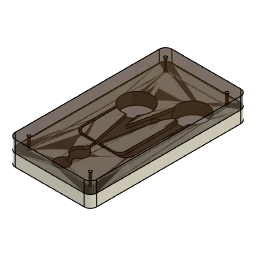
Exhaust_PEEP v7 (Autodesk Fusion 360 design; units mm, degrees)
Autodesk Fusion 360 part; units mm, degrees
sketch "Channels" plane through (0, 0, 0) normal (0, 0, 1) x (1, 0, 0)
  line L0 (0, 0) -> (46.5, 0)
  line L1 (46.5, 0) -> (46.5, 83)
  line L2 (46.5, 83) -> (0, 83)
  line L3 (0, 83) -> (0, 0)
  line L4 (27.5, -7) -> (27.5, 90) construction
  line L5 (10.6, 83) -> (10.6, 31.27) construction
  line L6 (46.5, 25.27) -> (16.6, 25.27) construction
  arc A0 (10.6, 31.27) -> (16.6, 25.27) centre (16.6, 31.27) ccw construction
  arc A1 (9.83, 31.27) -> (16.6, 24.5) centre (16.6, 31.27) ccw
  arc A2 (11.37, 31.27) -> (16.6, 26.04) centre (16.6, 31.27) ccw
  line L7 (27.5, 48.6) -> (34.1243, 80.3757)
  line L8 (27.5, 48.6) -> (46.5, 48.6) construction
  line L9 (27.5, 48.6) -> (25.0136, 60.5271)
  line L10 (25.8031, 26.04) -> (19.3855, 56.8243)
  line L11 (27.5, 17.9) -> (28.8759, 24.5) construction
  line L12 (29.1969, 26.04) -> (33.9, 48.6) construction
  line L13 (28.35, 24.5) -> (28.35, 21)
  line L14 (26.65, 24.5) -> (26.65, 21)
  arc A3 (28.35, 21) -> (30.6235, 17.0635) centre (32.8947, 21) ccw
  arc A4 (24.3765, 17.0635) -> (26.65, 21) centre (22.1053, 21) ccw
  line L15 (39.7, 26.04) -> (29.1969, 26.04)
  line L16 (25.8031, 26.04) -> (16.6, 26.04)
  line L17 (39.7, 24.5) -> (28.35, 24.5)
  line L18 (26.65, 24.5) -> (16.6, 24.5)
  line L19 (11.37, 57.9106) -> (11.37, 31.27)
  line L20 (9.83, 59.002) -> (9.83, 31.27)
  arc A5 (25.0136, 60.5271) -> (9.83, 59.002) centre (16.69, 67.05) ccw
  arc A6 (11.37, 57.9106) -> (19.3855, 56.8243) centre (16.69, 67.05) ccw
  circle A7 centre (16.69, 67.05) radius 7.5 construction
  line L21 (32.5, 0) -> (32.5, 7.9)
  line L22 (22.5, 0) -> (22.5, 7.9)
  arc A8 (24.3765, 17.0635) -> (22.5, 7.9) centre (27.5, 11.65) ccw
  arc A9 (22.5, 7.9) -> (27.5, 5.4) centre (27.5, 11.65) ccw construction
  arc A10 (27.5, 5.4) -> (32.5, 7.9) centre (27.5, 11.65) ccw construction
  arc A11 (32.5, 7.9) -> (30.6235, 17.0635) centre (27.5, 11.65) ccw
  line L23 (46.5, 29.62) -> (39.7, 29.62)
  line L24 (39.7, 20.92) -> (46.5, 20.92)
  line L25 (46.5, 20.92) -> (46.5, 29.62)
  line L26 (39.7, 29.62) -> (39.7, 26.04)
  line L27 (39.7, 24.5) -> (39.7, 20.92)
  line L28 (39.7, 25.27) -> (39.7, 24.5)
  line L29 (39.7, 26.04) -> (39.7, 25.27)
  arc A12 (41.7025, 72.7975) -> (36.748, 62.2613) centre (61.3232, 57.1381) ccw
  line L30 (29.1969, 26.04) -> (36.748, 62.2613)
  line L31 (39.4202, 75.0798) -> (41.0713, 83) construction
  line L32 (36.748, 62.2613) -> (39.4202, 75.0798) construction
  line L33 (46.5, 68) -> (41.7025, 72.7975)
  line L34 (34.1243, 80.3757) -> (31.5, 83)
  line L35 (39.4202, 75.0798) -> (34.1243, 80.3757)
  line L36 (41.7025, 72.7975) -> (39.4202, 75.0798)
  line L37 (34.1243, 80.3757) -> (34.6713, 83) construction
  line L38 (42.75, 29.62) -> (42.75, 71.75) construction
  arc A13 (30.6235, 17.0635) -> (27.5, 17.9) centre (27.5, 11.65) ccw construction
  arc A14 (24.3765, 17.0635) -> (30.6235, 17.0635) centre (27.5, 11.65) ccw
  arc A15 (27.5, 17.9) -> (24.3765, 17.0635) centre (27.5, 11.65) ccw construction
  circle A16 centre (16.69, 67.05) radius 11.125 construction
  dimension "d1" = 83
  dimension "d2" = 46.5
  dimension "d3" = 19
  dimension "d6" = 6
  dimension "d7" = 10.6
  dimension "d8" = 25.27
  dimension "d11" = 12.5
  dimension "d12" = 12.85
  dimension "d13" = 34.4
  dimension "d14" = 12.6
  dimension "d16" = 3.3939
  dimension "d17" = 0.85
  dimension "d20" = 21.15
  dimension "d21" = 16.69
  dimension "d22" = 15.95
  dimension "d23" = 0.77
  dimension "d24" = 0.77
  dimension "d25" = 11.776
  dimension "d26" = 15
  dimension "d27" = 5
  dimension "d28" = 8.7
  dimension "d29" = 6.8
  dimension "d30" = 15
  dimension "d31" = 15
  dimension "d32" = 37
  dimension "d33" = 2.7
  dimension "d34" = 1.54
  dimension "d35" = 1.7
  dimension "d36" = 6.2653
  dimension "d37" = 3.75
  dimension "d38" = 3.5
  dimension "d65" = 22.25
  constraint horizontal L0
  constraint vertical L1
  constraint horizontal L2
  constraint vertical L3
  constraint coincident L0.start L3.end
  constraint perpendicular L2 L4
  constraint perpendicular L2 L5
  constraint coincident L1 L6.start
  constraint coincident L5 L5.start
  constraint coincident L2 L5.start
  constraint tangent L6 A0
  constraint tangent L5 A0
  constraint coincident L4 A8.centre
  constraint coincident L4 L7.start
  constraint coincident L2 L37.end
  constraint coincident L4 L11.start
  constraint perpendicular L4 L8
  constraint coincident L12.end L8
  constraint coincident L2 L31.end
  constraint parallel L11 L30
  constraint parallel L7 L30
  constraint symmetric L4 L7.start L8.start
  constraint coincident L11.end L17
  constraint collinear L11 L12
  constraint coincident L10.start L15
  constraint perpendicular L13 L17
  constraint symmetric L4 L13.start L14.start
  constraint tangent L13 A3
  constraint coincident A3.end A8
  constraint symmetric L4 A3.end A4.start
  constraint symmetric L4 L13.end L14.end
  constraint symmetric L4 A3 A4
  constraint parallel L6 L15
  constraint concentric A0 A2
  constraint tangent A2 L15
  constraint collinear L15 L16
  constraint parallel L6 L17
  constraint concentric A0 A1
  constraint tangent A1 L17
  constraint collinear L17 L18
  constraint coincident A3 A11.end
  constraint coincident A4 A8.start
  constraint coincident L19.start A5
  constraint tangent A1 L20
  constraint concentric A5 A6
  constraint concentric A6 A7
  constraint coincident L1 L8.end
  constraint coincident L0 L21.start
  constraint coincident L21.end A8
  constraint perpendicular L0 L21
  constraint symmetric L4 L21.start L22.start
  constraint symmetric L4 L21.end L22.end
  constraint coincident L4 A9.end
  constraint concentric A8 A10
  constraint concentric A8 A9
  constraint concentric A10 A13
  constraint concentric A10 A11
  constraint horizontal L23
  constraint vertical L26
  constraint horizontal L24
  constraint vertical L25
  constraint coincident L1 L23.start
  constraint symmetric L6 L23 L24
  constraint coincident L17.start L26
  constraint coincident L6 L28.start
  constraint vertical L29
  constraint parallel L9 L10
  constraint coincident L1 L33.start
  constraint coincident L2 L34.end
  constraint tangent A12 L30
  constraint parallel L30 L37
  constraint collinear L33 L36
  constraint collinear L33 L34
  constraint coincident L33 L38.end
  constraint perpendicular L6 L38
  constraint coincident L23 L38.start
  constraint tangent A3 A11
  constraint concentric A13 A14
  constraint concentric A13 A15
  constraint concentric A5 A16
  measures "d1" distance of L0.start L2.end
  measures "d2" distance of L0.start L0.end
  measures "d3" horizontal distance of L0.end L4.start
  measures "d6" radius of A0
  measures "d7" distance of L3 L5
  measures "d8" distance of L0 L6
  measures "d11" diameter of A8
  measures "d12" distance of A8.centre L17
  measures "d13" distance of L2 L7.start
  measures "d14" distance of L1 L12.end
  measures "d16" distance of L12.start L10.start
  measures "d17" distance of L4 L13
  measures "d20" diameter of A5
  measures "d21" distance of L3 A5.centre
  measures "d22" distance of L2 A5.centre
  measures "d23" distance of L5 L19
  measures "d24" distance of L5 L20
  measures "d25" angle of L4 L7
  measures "d26" diameter of A7
  measures "d27" distance of L4 L21
  measures "d28" distance of L23.start L24.end
  measures "d29" distance of L23.start L23.end
  measures "d30" distance of L1.end L33.start
  measures "d31" distance of L1.end L34.end
  measures "d32" distance of L12.start A12.end
  measures "d33" distance of A12.start L30
  measures "d34" distance of L19 L20
  measures "d35" distance of L13 L14
  measures "d36" distance of L7 L30
  measures "d37" distance of L1 L38
  measures "d38" distance of L14.start L14.end
  measures "d65" diameter of A16
sketch "Body" plane through (0, 0, 0) normal (0, 0, 1) x (1, 0, 0)
  line L0 (27.5, -7) -> (27.5, 90) construction
  line L1 (27.5, 48.6) -> (34.1243, 80.3757) construction
  line L2 (29.1969, 26.04) -> (36.748, 62.2613) construction
  arc A0 (41.7025, 72.7975) -> (36.748, 62.2613) centre (61.3232, 57.1381) ccw construction
  line L3 (46.5, 25.27) -> (16.6, 25.27) construction
  circle A1 centre (16.4585, 68.1603) radius 11.7078
  line L4 (25.8031, 26.04) -> (19.3855, 56.8243) construction
  line L5 (19.3855, 56.8243) -> (16.4585, 70.8645) construction
  line L6 (16.4585, 68.1603) -> (15.5152, 72.6856) construction
  line L7 (30.5921, 48.0824) -> (38.9594, 88.2195) construction
  circle A2 centre (45.274, 83.9473) radius 11.7078
  circle A3 centre (45.2029, 25.27) radius 5.5565
  circle A4 centre (27.5, -2.35) radius 5.5565
  line L8 (39.7, 24.5) -> (28.35, 24.5) construction
  line L9 (-2.5, -14.7618) -> (62.5, -14.7618)
  line L10 (62.5, -14.7618) -> (62.5, 110.2382)
  line L11 (62.5, 110.2382) -> (-2.5, 110.2382)
  line L12 (-2.5, 110.2382) -> (-2.5, -14.7618)
  arc A5 (24.3765, 17.0635) -> (30.6235, 17.0635) centre (27.5, 11.65) ccw
  line L13 (25.5, 2.8341) -> (25.5, 5.7286)
  line L14 (29.5, 2.8341) -> (29.5, 5.7286)
  circle A6 centre (5.5, -6.7618) radius 1.1303
  circle A7 centre (54.5, 102.2382) radius 1.1303
  circle A8 centre (54.5, -6.7618) radius 1.1303
  circle A9 centre (5.5, 102.2382) radius 1.1303
  point P0 (27.5, 11.65)
  point P1 (16.69, 67.05)
  point P2 (19.3855, 56.8243)
  point P3 (41.7025, 72.7975)
  dimension "d78" = 23.4156
  dimension "d79" = 0.5519
  dimension "d82" = 6.2653
  dimension "d83" = 3.1327
  dimension "d84" = 23.4156
  dimension "d85" = 11.113
  dimension "d86" = 11.113
  dimension "d87" = 125
  dimension "d88" = 65
  dimension "d90" = 2
  dimension "d91" = 2
  dimension "d92" = 30
  dimension "d93" = 2.2606
  dimension "d94" = 2.2606
  dimension "d95" = 2.2606
  dimension "d96" = 2.2606
  dimension "d97" = 8
  dimension "d98" = 8
  dimension "d99" = 8
  dimension "d100" = 8
  dimension "d101" = 8
  dimension "d102" = 8
  dimension "d103" = 8
  dimension "d104" = 8
  dimension "d105" = 14
  constraint coincident P2 L4.end
  constraint parallel L4 L5
  constraint coincident A1.centre L6.start
  constraint parallel L5 L6
  constraint parallel L1 L7
  constraint coincident A2 P3
  constraint coincident L1.end A2
  constraint coincident A1 P2
  constraint coincident L3 A3.centre
  constraint coincident L0 A4.centre
  constraint coincident A3 L8.start
  constraint horizontal L9
  constraint vertical L10
  constraint horizontal L11
  constraint vertical L12
  constraint coincident A4 L13.start
  constraint coincident A5 L13.end
  constraint vertical L13
  constraint coincident A4 L14.start
  constraint coincident A5 L14.end
  constraint parallel L0 L14
  measures "d78" diameter of A1
  measures "d79" distance of L5 L6
  measures "d82" distance of L1 L2
  measures "d83" distance of L1 L7
  measures "d84" diameter of A2
  measures "d85" diameter of A3
  measures "d86" diameter of A4
  measures "d87" distance of L9 L11
  measures "d88" distance of L10 L12
  measures "d90" distance of L0 L13
  measures "d91" distance of L0 L14
  measures "d92" distance of L0 L12
  measures "d93" diameter of A6
  measures "d94" diameter of A7
  measures "d95" diameter of A8
  measures "d96" diameter of A9
  measures "d97" distance of L9 A6.centre
  measures "d98" distance of L12 A6.centre
  measures "d99" distance of L9 A8.centre
  measures "d100" distance of L10 A8.centre
  measures "d101" distance of L10 A7.centre
  measures "d102" distance of L11 A7.centre
  measures "d103" distance of L12 A9.centre
  measures "d104" distance of L11 A9.centre
  measures "d105" distance of A4.centre P0
sketch "Set screws" plane through (0, 0, 0) normal (0, 0, 1) x (1, 0, 0)
  line L0 (46.5, 25.27) -> (16.6, 25.27) construction
  line L1 (27.5, -7) -> (27.5, 90) construction
  arc A0 (10.6, 31.27) -> (16.6, 25.27) centre (16.6, 31.27) ccw construction
  line L2 (10.6, 83) -> (10.6, 31.27) construction
  circle A1 centre (33, 25.27) radius 1.1303
  circle A2 centre (10.6, 40.27) radius 1.1303
  line L3 (27.5, 48.6) -> (34.1243, 80.3757) construction
  line L4 (29.1969, 26.04) -> (36.748, 62.2613) construction
  line L5 (29.3106, 41.9352) -> (35.5849, 72.0324) construction
  circle A3 centre (34.244, 65.6) radius 2.7051
  line L6 (27.5, 48.6) -> (46.5, 48.6)
  dimension "d61" = 2.2606
  dimension "d62" = 2.2606
  dimension "d63" = 5.5
  dimension "d64" = 15
  dimension "d106" = 6.2653
  dimension "d107" = 3.1327
  dimension "d108" = 5.4102
  dimension "d109" = 17
  constraint coincident L0 A1.centre
  constraint coincident L2 A2.centre
  constraint parallel L4 L5
  constraint coincident L5 A3.centre
  measures "d61" diameter of A1
  measures "d62" diameter of A2
  measures "d63" distance of L1 A1.centre
  measures "d64" distance of L0 A2.centre
  measures "d106" distance of L3 L4
  measures "d107" distance of L3 L5
  measures "d108" diameter of A3
  measures "d109" distance of A3.centre L6
sketch "Side channel" plane through (0, 0, 0) normal (0, 0, 1) x (1, 0, 0)
  line L0 (39.7, 24.5) -> (28.35, 24.5)
  line L1 (39.7, 26.04) -> (29.1969, 26.04)
  circle A0 centre (45.274, 83.9473) radius 11.7078
  line L2 (45.0545, 72.2415) -> (45.0545, 31.04)
  line L3 (40.0545, 26.04) -> (39.7, 26.04)
  line L4 (39.7, 24.5) -> (45.5545, 24.5)
  line L5 (51.5545, 30.5) -> (51.5545, 74.0666)
  arc A1 (40.0545, 26.04) -> (45.0545, 31.04) centre (40.0545, 31.04) ccw
  arc A2 (45.5545, 24.5) -> (51.5545, 30.5) centre (45.5545, 30.5) ccw
  line L6 (39.7, 26.04) -> (39.7, 24.5)
  dimension "d123" = 5
  dimension "d124" = 6
  dimension "d125" = 6.5
  constraint coincident A0 L2.start
  constraint vertical L2
  constraint coincident L1.start L3.end
  constraint coincident L0.start L4.start
  constraint perpendicular L2 L4
  constraint coincident A0 L5.end
  constraint perpendicular L4 L5
  constraint horizontal L3
  constraint tangent L2 A1
  constraint tangent L3 A1
  constraint tangent L5 A2
  constraint tangent L4 A2
  measures "d123" radius of A1
  measures "d124" radius of A2
  measures "d125" distance of L2 L5
extrude "Extrude10" add sketch "Body" along normal blind 9.525 and the other way blind 9.525 contours A1 | A2 | A3 | A4 | A4 A5 L13 L14 | L9 L10 L11 L12 | A6 | A7 | A8 | A9 makes body 1
extrude "Extrude11" cut sketch "Channels" against normal blind 2.25 contours A1 L7 L9 L13 L14 A3 A4 L15 L17 L18 L20 A5 A8 A11 L28 L29 A12 L30 L35 L36 A14 bodies 1
extrude "Extrude16" cut sketch "Side channel" against normal blind 2.25 contours A0 L2 L3 L4 L5 A1 A2 L6 bodies 1
extrude "Extrude12" cut sketch "Body" against normal through all contours A1 | A2 | A4 bodies 1
extrude "Extrude13" cut sketch "Set screws" against normal through all bodies 1
extrude "Extrude15" cut sketch "Body" against normal blind 2.25 contours A4 A5 L13 L14 bodies 1
extrude "Extrude14" cut sketch "Body" along normal through all and the other way through all contours A6 | A7 | A8 | A9 bodies 1
fillet "Fillet3" radius 5 4 edges at (62.5, -14.7618, 0) (-2.5, -14.7618, 0) (62.5, 110.2382, 0) (-2.5, 110.2382, 0) on bodies 1
split "Split2" by plane through (0, 0, 0) normal (0, 0, 1) bodies 1 makes body 2 at (21.9669, 65.5526, 9.525)
equation "d12 = ( 12.5 / 2 ) * 1 mm + 6.60 mm"
equation "d83 = 6.265305 mm / 2"
equation "d84 = d78"
equation "d94 = d93"
equation "d95 = d93"
equation "d96 = d93"
equation "d98 = d97"
equation "d99 = d97"
equation "d100 = d97"
equation "d101 = d97"
equation "d102 = d97"
equation "d103 = d97"
equation "d104 = d97"
equation "d107 = 6.265305 mm / 2"
named bodies: "Base", "Cover"
